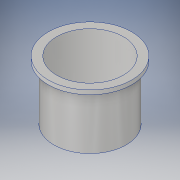
# Autodesk Inventor part: Aluminum Carrier 8-inch v1
Saved by Autodesk Inventor 2017 (Build 210142000, 142)
## iProperties
Created: 2016-07-07
Part Number: Aluminum Carrier 8-inch v1
Material: Aluminum 6061
Document SubType Name: Modeling
Designer: Bill
Density: 2.7 g/cm^3
Appearance: Aluminum - Flat
Author: Bill
Autodesk Inventor part; units mm, degrees
ref_plane "YZ Plane" through (0, 0, 0) normal (1, 0, 0) x (0, 1, 0)
ref_plane "XZ Plane" through (0, 0, 0) normal (0, 1, 0) x (-1, 0, 0)
ref_plane "XY Plane" through (0, 0, 0) normal (0, 0, 1) x (1, 0, 0)
sketch "Sketch1" plane through (0, 0, 0) normal (0, 0, 1) x (1, 0, 0)
  line L0 (0, 0) -> (0, 42.0297) construction
  line L1 (-76.2, 18.4955) -> (-95.25, 18.4955)
  line L2 (-95.25, 18.4955) -> (-95.25, 8.9705)
  line L3 (-95.25, 8.9705) -> (-82.55, 8.9705)
  line L4 (-82.55, 8.9705) -> (-82.55, -116.3277)
  line L5 (-82.55, -116.3277) -> (-76.2, -116.3277)
  line L6 (-69.85, -92.6295) -> (-76.2, -92.6295)
  line L7 (-76.2, 18.4955) -> (-76.2, -92.6295)
  line L8 (-69.85, -92.6295) -> (-76.2, -116.3277)
  dimension "d2" = 19.05
  dimension "d3" = 9.525
  dimension "d4" = 125.2982
  dimension "d6" = 12.7
  dimension "d7" = 6.35
  dimension "d8" = 6.35
  dimension "d9" = 95.25
  dimension "d11" = 111.125
  constraints: 18 end point, 4 perpendicular, 2 horizontal, 2 vertical
  measures "d2" distance of L1.start L1.end
  measures "d3" distance of L1.end L2.end
  measures "d4" distance of L3.end L4.end
  measures "d6" distance of L2.end L3.end
  measures "d7" distance of L4.end L5.end
  measures "d8" distance of L6.start L6.end
  measures "d9" distance from line of L0 L1.end
  measures "d11" distance of L1.start L6.end
revolve "Revolution1" add sketch "Sketch1" angle 360 about axis through (0, 0, 0) along (0, 1, 0)
body "Solid1"
